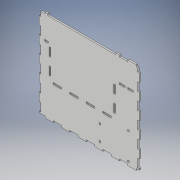
# Autodesk Inventor part: 5 onder plaat
Saved by Autodesk Inventor 2019 (Build 230136000, 136)
## iProperties
Created: 2021-01-09
Part Number: 5 onder plaat
Material: Generic
Document SubType Name: Sheet Metal
Designer: Stefan
Density: 1 g/cm^3
Sheet Metal Rule: Default_mm
Appearance: Default
Author: Stefan
Autodesk Inventor part; units mm, degrees
ref_plane "YZ Plane" through (0, 0, 0) normal (1, 0, 0) x (0, 1, 0)
ref_plane "XZ Plane" through (0, 0, 0) normal (0, 1, 0) x (-1, 0, 0)
ref_plane "XY Plane" through (0, 0, 0) normal (0, 0, 1) x (1, 0, 0)
sketch "Sketch1" plane through (0, 0, 0) normal (0, 0, 1) x (1, 0, 0)
  line L0 (-70, -65) -> (70, -65)
  line L1 (-70, 65) -> (-70, -65)
  line L2 (-70, -65) -> (70, 65) construction
  line L3 (70, -65) -> (-70, 65) construction
  line L4 (-52.5, -18) -> (-37.5, -18)
  line L5 (-37.5, -18) -> (-37.5, -15)
  line L6 (-37.5, -15) -> (-52.5, -15)
  line L7 (-52.5, -15) -> (-52.5, -18)
  line L8 (-52.5, -18) -> (-37.5, -15) construction
  line L9 (-37.5, -18) -> (-52.5, -15) construction
  line L10 (-22.5, -18) -> (-7.5, -18)
  line L11 (-7.5, -18) -> (-7.5, -15)
  line L12 (-7.5, -15) -> (-22.5, -15)
  line L13 (-22.5, -15) -> (-22.5, -18)
  line L14 (-22.5, -18) -> (-7.5, -15) construction
  line L15 (-7.5, -18) -> (-22.5, -15) construction
  line L16 (7.5, -18) -> (22.5, -18)
  line L17 (22.5, -18) -> (22.5, -15)
  line L18 (22.5, -15) -> (7.5, -15)
  line L19 (7.5, -15) -> (7.5, -18)
  line L20 (7.5, -18) -> (22.5, -15) construction
  line L21 (22.5, -18) -> (7.5, -15) construction
  line L22 (37.5, -18) -> (52.5, -18)
  line L23 (52.5, -18) -> (52.5, -15)
  line L24 (52.5, -15) -> (37.5, -15)
  line L25 (37.5, -15) -> (37.5, -18)
  line L26 (37.5, -18) -> (52.5, -15) construction
  line L27 (52.5, -18) -> (37.5, -15) construction
  line L28 (-52.5, -15) -> (-57, -15) construction
  line L29 (-57, -15) -> (-57, -7.5) construction
  line L30 (-57, -7.5) -> (-60, -7.5)
  line L31 (-60, -7.5) -> (-60, 7.5)
  line L32 (-60, 7.5) -> (-57, 7.5)
  line L33 (-57, 7.5) -> (-57, -7.5)
  line L34 (-60, 37.5) -> (-57, 37.5)
  line L35 (-60, 22.5) -> (-60, 37.5)
  line L36 (-57, 37.5) -> (-57, 22.5)
  line L37 (-57, 22.5) -> (-60, 22.5)
  line L38 (57, 7.5) -> (60, 7.5)
  line L39 (57, -7.5) -> (57, 7.5)
  line L40 (60, 7.5) -> (60, -7.5)
  line L41 (60, -7.5) -> (57, -7.5)
  line L42 (57, 37.5) -> (60, 37.5)
  line L43 (57, 22.5) -> (57, 37.5)
  line L44 (60, 37.5) -> (60, 22.5)
  line L45 (60, 22.5) -> (57, 22.5)
  line L46 (70, -65) -> (100, -65)
  line L47 (100, -65) -> (100, 85)
  line L48 (100, 85) -> (-70, 85)
  line L49 (-70, 85) -> (-70, 65)
  point P0 (0, 0)
  point P1 (-45, -16.5)
  point P2 (-15, -16.5)
  point P3 (15, -16.5)
  point P4 (45, -16.5)
  dimension "d0" = 140
  dimension "d1" = 130
  dimension "d2" = 15
  dimension "d3" = 3
  dimension "d4" = 17.5
  dimension "d8" = 30
  dimension "d13" = 4.5
  dimension "d14" = 7.5
  dimension "d15" = 3
  dimension "d16" = 15
  dimension "d19" = 30
  dimension "d22" = 117
  dimension "d27" = 30
  dimension "d28" = 150
  dimension "d29" = 47.121
  dimension "d30" = 47.121
  dimension "d31" = 57.5
  constraints: 100 end point, 10 midpoint, 6 perpendicular, 5 horizontal, 5 parallel, 3 collinear, 1 point on line, 1 vertical, 54 other
  measures "d0" distance of L1.start L2.end
  measures "d1" distance of L2.end L0.end
  measures "d2" distance of L6.end L5.end
  measures "d3" distance of L5.end L4.end
  measures "d4" distance between parallel lines of L7 L1
  measures "d8" distance of L4.start L10.start
  measures "d13" distance of L6.end L28.end
  measures "d14" distance of L28.end L29.end
  measures "d15" distance of L31.end L32.end
  measures "d16" distance of L30.end L31.end
  measures "d19" distance of L31.end L34.start
  measures "d22" distance of L31.end L38.start
  measures "d27" distance of L0.end L46.end
  measures "d28" distance of L46.end L47.end
  measures "d29" angle of L47 L2
  measures "d30" angle of L47 L3
  measures "d31" distance between parallel lines of L30 L46
extrude "Extrusion1" add sketch "Sketch1" along normal blind 3
sketch "Sketch2" plane through (0, 0, 3) normal (0, 0, 1) x (1, 0, 0)
  line L0 (100, 85) -> (-70, 85) projected
  line L1 (-67.5, 85) -> (-52.5, 85)
  line L2 (-52.5, 85) -> (-52.5, 88)
  line L3 (-52.5, 88) -> (-67.5, 88)
  line L4 (-67.5, 88) -> (-67.5, 85)
  line L5 (-70, 85) -> (-70, -65) projected
  line L6 (-37.5, 85) -> (-22.5, 85)
  line L7 (-22.5, 85) -> (-22.5, 88)
  line L8 (-22.5, 88) -> (-37.5, 88)
  line L9 (-37.5, 88) -> (-37.5, 85)
  line L10 (-7.5, 85) -> (7.5, 85)
  line L11 (7.5, 85) -> (7.5, 88)
  line L12 (7.5, 88) -> (-7.5, 88)
  line L13 (-7.5, 88) -> (-7.5, 85)
  line L14 (22.5, 85) -> (37.5, 85)
  line L15 (37.5, 85) -> (37.5, 88)
  line L16 (37.5, 88) -> (22.5, 88)
  line L17 (22.5, 88) -> (22.5, 85)
  line L18 (52.5, 85) -> (67.5, 85)
  line L19 (67.5, 85) -> (67.5, 88)
  line L20 (67.5, 88) -> (52.5, 88)
  line L21 (52.5, 88) -> (52.5, 85)
  line L22 (82.5, 85) -> (97.5, 85)
  line L23 (97.5, 85) -> (97.5, 88)
  line L24 (97.5, 88) -> (82.5, 88)
  line L25 (82.5, 88) -> (82.5, 85)
  line L26 (-67.5, -78) -> (-52.5, -78)
  line L27 (-52.5, -78) -> (-52.5, -75)
  line L28 (-52.5, -75) -> (-67.5, -75)
  line L29 (-67.5, -75) -> (-67.5, -78)
  line L30 (-37.5, -78) -> (-22.5, -78)
  line L31 (-22.5, -78) -> (-22.5, -75)
  line L32 (-22.5, -75) -> (-37.5, -75)
  line L33 (-37.5, -75) -> (-37.5, -78)
  line L34 (-7.5, -78) -> (7.5, -78)
  line L35 (7.5, -78) -> (7.5, -75)
  line L36 (7.5, -75) -> (-7.5, -75)
  line L37 (-7.5, -75) -> (-7.5, -78)
  line L38 (22.5, -78) -> (37.5, -78)
  line L39 (37.5, -78) -> (37.5, -75)
  line L40 (37.5, -75) -> (22.5, -75)
  line L41 (22.5, -75) -> (22.5, -78)
  line L42 (52.5, -78) -> (67.5, -78)
  line L43 (67.5, -78) -> (67.5, -75)
  line L44 (67.5, -75) -> (52.5, -75)
  line L45 (52.5, -75) -> (52.5, -78)
  line L46 (82.5, -78) -> (97.5, -78)
  line L47 (97.5, -78) -> (97.5, -75)
  line L48 (97.5, -75) -> (82.5, -75)
  line L49 (82.5, -75) -> (82.5, -78)
  line L50 (-70, 77.5) -> (-73, 77.5)
  line L51 (-73, 77.5) -> (-73, 62.5)
  line L52 (-73, 62.5) -> (-70, 62.5)
  line L53 (-70, 62.5) -> (-70, 77.5)
  line L54 (-70, 32.5) -> (-70, 47.5)
  line L55 (-73, 32.5) -> (-70, 32.5)
  line L56 (-73, 47.5) -> (-73, 32.5)
  line L57 (-70, 47.5) -> (-73, 47.5)
  line L58 (-70, 2.5) -> (-70, 17.5)
  line L59 (-73, 2.5) -> (-70, 2.5)
  line L60 (-73, 17.5) -> (-73, 2.5)
  line L61 (-70, 17.5) -> (-73, 17.5)
  line L62 (-70, -27.5) -> (-70, -12.5)
  line L63 (-73, -27.5) -> (-70, -27.5)
  line L64 (-73, -12.5) -> (-73, -27.5)
  line L65 (-70, -12.5) -> (-73, -12.5)
  line L66 (-70, -57.5) -> (-70, -42.5)
  line L67 (-73, -57.5) -> (-70, -57.5)
  line L68 (-73, -42.5) -> (-73, -57.5)
  line L69 (-70, -42.5) -> (-73, -42.5)
  line L70 (103, 62.5) -> (103, 77.5)
  line L71 (100, 62.5) -> (103, 62.5)
  line L72 (100, 77.5) -> (100, 62.5)
  line L73 (103, 77.5) -> (100, 77.5)
  line L74 (103, 32.5) -> (103, 47.5)
  line L75 (100, 32.5) -> (103, 32.5)
  line L76 (100, 47.5) -> (100, 32.5)
  line L77 (103, 47.5) -> (100, 47.5)
  line L78 (103, 2.5) -> (103, 17.5)
  line L79 (100, 2.5) -> (103, 2.5)
  line L80 (100, 17.5) -> (100, 2.5)
  line L81 (103, 17.5) -> (100, 17.5)
  line L82 (103, -27.5) -> (103, -12.5)
  line L83 (100, -27.5) -> (103, -27.5)
  line L84 (100, -12.5) -> (100, -27.5)
  line L85 (103, -12.5) -> (100, -12.5)
  line L86 (103, -57.5) -> (103, -42.5)
  line L87 (100, -57.5) -> (103, -57.5)
  line L88 (100, -42.5) -> (100, -57.5)
  line L89 (103, -42.5) -> (100, -42.5)
  point P0 (0, 0)
  dimension "d32" = 15
  dimension "d33" = 3
  dimension "d34" = 2.5
  dimension "d37" = 30
  dimension "d40" = 163
  dimension "d43" = 3
  dimension "d44" = 15
  dimension "d45" = 7.5
  dimension "d48" = 30
  dimension "d51" = 173
  dimension "d138" = 15
  dimension "d139" = 37.5
  constraints: 176 end point, 4 horizontal, 4 parallel, 2 perpendicular, 2 point on line, 2 vertical, 160 other
  measures "d32" distance of L3.end L2.end
  measures "d33" distance of L2.end L1.end
  measures "d34" distance between parallel lines of L5 L4
  measures "d37" distance of L1.start L6.start
  measures "d40" distance of L1.start L26.start
  measures "d43" distance of L52.end L51.end
  measures "d44" distance of L51.end L50.end
  measures "d45" distance from line of L0.end L50
  measures "d48" distance of L50.start L54.end
  measures "d51" distance of L50.start L70.end
  measures "d138" distance between parallel lines of L55 L61
  measures "d139" vertical distance of L0.end L56.start
extrude "Extrusion2" add sketch "Sketch2" against normal blind 3
sketch "Sketch3" plane through (0, 0, 3) normal (0, 0, 1) x (1, 0, 0)
  line L0 (-57, 22.5) -> (-57, 37.5) projected
  line L1 (-70, 62.5) -> (-70, 47.5) projected
  line L2 (-73, 32.5) -> (-73, 47.5) projected
  line L3 (-62, 42) -> (-62, 45)
  line L4 (-62, 45) -> (-68, 45)
  line L5 (-68, 45) -> (-68, 42)
  line L6 (-68, 42) -> (-62, 42)
  line L7 (-60, 37.5) -> (-60, 22.5) construction
  line L8 (-60, 37.5) -> (-60, 42) construction
  line L9 (-60, 42) -> (-62, 42) construction
  point P0 (0, 0)
  dimension "d67" = 3
  dimension "d68" = 6
  dimension "d69" = 4.5
  dimension "d70" = 2
  constraints: 12 end point, 4 perpendicular, 2 vertical
  measures "d67" distance of L3.start L3.end
  measures "d68" distance of L3.end L4.end
  measures "d69" distance of L7.start L8.end
  measures "d70" distance of L8.end L3.start
extrude "Extrusion3" cut sketch "Sketch3" against normal blind 3
sketch "Sketch4" plane through (0, 0, 3) normal (0, 0, 1) x (1, 0, 0)
  line L0 (57, 37.5) -> (57, 22.5) projected
  line L1 (60, 37.5) -> (60, 42) construction
  line L2 (100, 47.5) -> (100, 62.5) projected
  line L3 (-62, 42) -> (-62, 45) projected
  line L4 (60, 42) -> (67.5, 42) construction
  line L5 (67.5, 42) -> (77.5, 42)
  line L6 (77.5, 42) -> (77.5, 45)
  line L7 (77.5, 45) -> (67.5, 45)
  line L8 (67.5, 45) -> (67.5, 42)
  line L9 (77.5, 42) -> (82.5, 42) construction
  line L10 (82.5, 42) -> (92.5, 42)
  line L11 (92.5, 42) -> (92.5, 45)
  line L12 (92.5, 45) -> (82.5, 45)
  line L13 (82.5, 45) -> (82.5, 42)
  point P0 (0, 0)
  dimension "d75" = 4.5
  dimension "d81" = 7.5
  dimension "d82" = 10
  dimension "d83" = 3
  dimension "d84" = 5
  dimension "d85" = 10
  dimension "d86" = 3
  constraints: 22 end point, 4 horizontal, 4 parallel, 2 perpendicular, 1 vertical
  measures "d75" distance of L1.start L1.end
  measures "d81" distance of L1.end L4.end
  measures "d82" distance of L7.end L6.end
  measures "d83" distance of L6.end L5.end
  measures "d84" distance of L5.end L9.end
  measures "d85" distance of L12.end L11.end
  measures "d86" distance of L11.end L10.end
extrude "Extrusion4" cut sketch "Sketch4" against normal blind 3
sketch "Sketch5" plane through (0, 0, 3) normal (0, 0, 1) x (1, 0, 0)
  line L0 (-70, 85) -> (-70, 77.5) projected
  line L1 (-70, 85) -> (-75, 85)
  line L2 (-75, 85) -> (-75, 77.5)
  line L3 (-75, 77.5) -> (-78, 77.5)
  line L4 (-78, 77.5) -> (-78, 62.5)
  line L5 (-78, 62.5) -> (-75, 62.5)
  line L6 (-75, 62.5) -> (-75, 47.5)
  line L7 (-75, 47.5) -> (-78, 47.5)
  line L8 (-78, 47.5) -> (-78, 32.5)
  line L9 (-78, 32.5) -> (-75, 32.5)
  line L10 (-75, 32.5) -> (-75, 17.5)
  line L11 (-75, 17.5) -> (-78, 17.5)
  line L12 (-78, 17.5) -> (-78, 2.5)
  line L13 (-78, 2.5) -> (-75, 2.5)
  line L14 (-75, 2.5) -> (-75, -12.5)
  line L15 (-75, -12.5) -> (-78, -12.5)
  line L16 (-78, -12.5) -> (-78, -27.5)
  line L17 (-78, -27.5) -> (-75, -27.5)
  line L18 (-75, -27.5) -> (-75, -42.5)
  line L19 (-75, -42.5) -> (-78, -42.5)
  line L20 (-78, -42.5) -> (-78, -57.5)
  line L21 (-78, -57.5) -> (-75, -57.5)
  line L22 (-75, -57.5) -> (-75, -65)
  line L23 (-70, -65) -> (100, -65) projected
  line L24 (-75, -65) -> (-70, -65)
  line L25 (-70, -65) -> (-70, 85)
  point P0 (0, 0)
  point P1 (-67.5, -65)
  dimension "d89" = 5
  dimension "d90" = 7.5
  dimension "d91" = 3
  dimension "d92" = 15
  dimension "d93" = 3
  dimension "d94" = 15
  dimension "d95" = 3
  dimension "d96" = 15
  dimension "d97" = 3
  dimension "d98" = 15
  dimension "d99" = 3
  dimension "d100" = 15
  dimension "d101" = 3
  dimension "d102" = 15
  dimension "d103" = 3
  dimension "d104" = 15
  dimension "d105" = 3
  dimension "d106" = 15
  dimension "d107" = 3
  dimension "d108" = 15
  dimension "d109" = 3
  dimension "d110" = 7.5
  constraints: 48 end point, 18 point on line, 7 parallel, 5 perpendicular, 1 horizontal
  measures "d89" distance of L0.start L1.end
  measures "d90" distance of L1.end L2.end
  measures "d91" distance of L2.end L3.end
  measures "d92" distance of L3.end L4.end
  measures "d93" distance of L4.end L5.end
  measures "d94" distance of L5.end L6.end
  measures "d95" distance of L6.end L7.end
  measures "d96" distance of L7.end L8.end
  measures "d97" distance of L8.end L9.end
  measures "d98" distance of L9.end L10.end
  measures "d99" distance of L10.end L11.end
  measures "d100" distance of L11.end L12.end
  measures "d101" distance of L12.end L13.end
  measures "d102" distance of L13.end L14.end
  measures "d103" distance of L14.end L15.end
  measures "d104" distance of L15.end L16.end
  measures "d105" distance of L16.end L17.end
  measures "d106" distance of L17.end L18.end
  measures "d107" distance of L18.end L19.end
  measures "d108" distance of L19.end L20.end
  measures "d109" distance of L20.end L21.end
  measures "d110" distance of L21.end L22.end
extrude "Extrusion5" add sketch "Sketch5" against normal blind 3
sketch "Sketch6" plane through (0, 0, 0) normal (0, 0, -1) x (-1, 0, 0)
  line L0 (-103, 88) -> (-60.2, 88) construction
  line L1 (-52.5, 88) -> (-67.5, 88) projected
  line L2 (-60.2, 88) -> (-60.2, 85)
  line L3 (78, 85) -> (62.7, 85) construction
  line L4 (67.5, 85) -> (75, 85) projected
  line L5 (62.7, 85) -> (62.7, 88)
  line L6 (67.5, 88) -> (52.5, 88) projected
  line L7 (62.7, 85) -> (-60.2, 85)
  line L8 (-60.2, 88) -> (62.7, 88)
  point P0 (0, 0)
  dimension "d113" = 42.8
  dimension "d114" = 3
  dimension "d115" = 15.3
  dimension "d116" = 122.9
  dimension "d117" = 12.3
  constraints: 12 end point, 3 perpendicular, 2 collinear, 2 point on line, 1 parallel
  measures "d113" distance of L0.start L0.end
  measures "d114" distance of L0.end L2.end
  measures "d115" distance of L3.start L3.end
  measures "d116" distance between parallel lines of L5 L2
  measures "d117" distance from line of L4.end L5
extrude "Extrusion6" cut sketch "Sketch6" against normal blind 3
sketch "Sketch9" plane through (0, 0, 3) normal (0, 0, 1) x (1, 0, 0)
  line L0 (-75, -65) -> (100, -65) projected
  line L1 (-75, -65) -> (100, -65)
  line L2 (100, -65) -> (100, -75)
  line L3 (100, -75) -> (-75, -75)
  line L4 (-75, -75) -> (-75, -65)
  line L5 (-78, -57.5) -> (-75, -57.5) construction
  line L6 (-78, -57.5) -> (-78, -72.5) construction
  line L7 (-78, -72.5) -> (-75, -72.5)
  line L8 (-75, -72.5) -> (-75, -75)
  line L9 (-75, -75) -> (-78, -75)
  line L10 (-78, -75) -> (-78, -72.5)
  line L11 (100, -75) -> (103, -75)
  line L12 (103, -75) -> (103, -72.5)
  line L13 (103, -72.5) -> (100, -72.5)
  line L14 (100, -72.5) -> (100, -75)
  point P0 (0, 0)
  dimension "d140" = 175
  dimension "d141" = 10
  dimension "d143" = 15
  dimension "d144" = 3
  dimension "d145" = 2.5
  constraints: 26 end point, 6 parallel, 3 horizontal, 3 perpendicular, 1 vertical
  measures "d140" distance of L2.end L3.end
  measures "d141" distance of L1.end L2.end
  measures "d143" distance of L5.start L6.end
  measures "d144" distance of L13.end L12.end
  measures "d145" distance of L12.end L11.end
extrude "Extrusion9" add sketch "Sketch9" against normal blind 3
sketch "Sketch10" plane through (0, 0, 0) normal (0, 0, -1) x (-1, 0, 0)
  circle A0 centre (-32.05, -65.5) radius 1.75
  line L0 (-29.3, -73.25) -> (-29.3, -19.75) construction
  circle A1 centre (-32.05, -37.5) radius 1.75
  line L1 (-29.3, -19.75) -> (-98, -19.75) construction
  line L2 (-98, -73.25) -> (-29.3, -73.25) construction
  line L3 (-29.3, -19.75) -> (-98, -73.25) construction
  line L4 (-98, -19.75) -> (-29.3, -73.25) construction
  circle A2 centre (-83.75, -22.5) radius 1.75
  line L5 (-98, -19.75) -> (-98, -73.25) construction
  circle A3 centre (-83.75, -70.5) radius 1.75
  line L6 (-84.5, -75) -> (-69.5, -75)
  line L7 (-39.5, -18) -> (-54.5, -18)
  line L8 (-100, -57.5) -> (-100, -72.5)
  line L9 (-100, -57.5) -> (-100, -72.5) projected
  point P0 (0, 0)
  point P1 (0, 0)
  point P2 (-63.65, -46.5)
  dimension "d148" = 68.7
  dimension "d149" = 53.5
  dimension "d150" = 3.5
  dimension "d151" = 1
  dimension "d152" = 12.5
  dimension "d153" = 3.5
  dimension "d154" = 1
  dimension "d155" = 12.5
  dimension "d156" = 3.5
  dimension "d157" = 1
  dimension "d158" = 3.5
  dimension "d159" = 1
  dimension "d160" = 6
  dimension "d161" = 16
  dimension "d162" = 1.75
  dimension "d163" = 1.75
  dimension "d164" = 2
  dimension "d165" = 1.75
  dimension "d170" = 10.2
  dimension "d171" = 25.2
  dimension "d172" = 40.2
  dimension "d173" = 55.2
  dimension "d174" = 39.5
  dimension "d175" = 54.5
  dimension "d178" = 0
  dimension "d179" = 18
  dimension "d180" = 100
  dimension "d181" = 18
  constraints: 18 end point, 4 centre point, 2 midpoint, 2 parallel, 1 perpendicular, 1 vertical
  measures "d148" distance of L4.end L5.end
  measures "d149" distance of L5.end L5.start
  measures "d150" diameter of A3
  measures "d151" distance edge to line of A3 L2
  measures "d152" distance edge to line of A3 L5
  measures "d153" diameter of A2
  measures "d154" distance edge to line of A2 L1
  measures "d155" distance edge to line of A2 L5
  measures "d156" diameter of A0
  measures "d157" distance edge to line of A0 L0
  measures "d158" diameter of A1
  measures "d159" distance edge to line of A1 L0
  measures "d160" distance edge to line of A0 L2
  measures "d161" distance edge to line of A1 L1
  measures "d162" distance between parallel lines of L6 L2
  measures "d163" distance between parallel lines of L7 L1
  measures "d164" distance between parallel lines of L5 L8
  measures "d165" distance between parallel lines of L7 L1
  measures "d170" distance from line of L7.start L0
  measures "d171" distance from line of L7.end L0
  measures "d172" distance from line of L6.end L0
  measures "d173" distance from line of L6.start L0
  measures "d174" distance from line of L8.start L7
  measures "d175" distance from line of L8.end L7
  measures "d178" distance between parallel lines of L9 L8
  measures "d179" distance from line of point (0, 0) L7
  measures "d180" distance from line of point (0, 0) L9
  measures "d181" distance from line of point (0, 0) L7
extrude "Extrusion10" cut sketch "Sketch10" against normal blind 10
equation "\"d150\" = d153"
equation "\"d156\" = d153"
equation "\"d158\" = d153"
equation "\"d162\" = d163"
equation "\"BendRadius\" = Thickness"
equation "\"BendReliefWidth\" = Thickness"
equation "\"BendReliefDepth\" = 0.5 * Thickness"
equation "\"CornerReliefSize\" = 4 * Thickness"
equation "\"MinimumRemnant\" = 2 * Thickness"
equation "\"TransitionRadius\" = BendRadius"
equation "\"JacobiRadiusSize\" = BendRadius"
equation "\"GapSize\" = Thickness"
equation "\"Thickness\" = 0.5"
body "Solid1"
